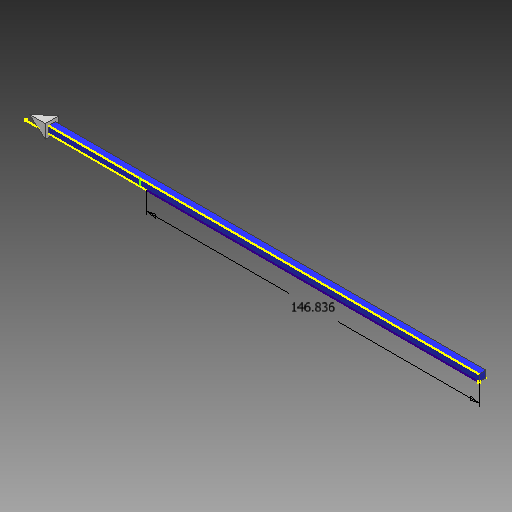
# Autodesk Inventor part: blueStick
Saved by Autodesk Inventor 2018.2 (Build 222227000, 227)
## iProperties
Created: 2018-04-12
Part Number: blueStick
Material: Generisch
Document SubType Name: Modeling
Designer: Nick Koch
Density: 1 g/cm^3
Appearance: Vorgabe
Author: Nick Koch
Autodesk Inventor part; units mm, degrees
ref_plane "YZ Plane" through (0, 0, 0) normal (1, 0, 0) x (0, 1, 0)
ref_plane "XZ Plane" through (0, 0, 0) normal (0, 1, 0) x (-1, 0, 0)
ref_plane "XY Plane" through (0, 0, 0) normal (0, 0, 1) x (1, 0, 0)
sketch "Skizze1" plane through (0, 0, 0) normal (0, 0, 1) x (1, 0, 0)
  line L0 (0, 0) -> (200, 0)
  line L1 (200, 0) -> (200, 3)
  line L2 (200, 3) -> (0, 3)
  line L3 (0, 3) -> (0, 0)
  dimension "d0" = 200
  dimension "d1" = 3
  constraints: 8 end point, 2 parallel, 1 horizontal, 1 perpendicular
  measures "d0" distance of L2.end L1.end
  measures "d1" distance of L1.end L0.end
extrude "Extrusion1" add sketch "Skizze1" along normal blind 3
sketch "Skizze2" plane through (200, 0, 0) normal (1, 0, 0) x (0, 0, -1)
  point P0 (0, 0)
sketch "Skizze3" plane through (0, 0, 0) normal (0, -1, 0) x (1, 0, 0)
  line L0 (0, 0) -> (200, 0) projected
  line L1 (200, 0) -> (53.164, 0)
  dimension "d4" = 146.836
  constraints: 2 end point, 1 point on line
  measures "d4" distance of L0.end L1.end
sketch "Skizze4" plane through (10, 0, 0) normal (-1, 0, 0) x (0, 0, 1)
  line L0 (0, 3) -> (3, 3) projected
  line L1 (0, 0) -> (3, 3)
  line L2 (3, 3) -> (0, 3)
  line L3 (0, 3) -> (3, 0)
  line L4 (-1.5, -1.5) -> (4.5, -1.5)
  line L5 (4.5, -1.5) -> (4.5, 4.5)
  line L6 (4.5, 4.5) -> (-1.5, 4.5)
  line L7 (-1.5, 4.5) -> (-1.5, -1.5)
  line L8 (-1.5, -1.5) -> (4.5, 4.5) construction
  line L9 (4.5, -1.5) -> (-1.5, 4.5) construction
  point P0 (1.5, 1.5)
  dimension "d14" = 6
  dimension "d15" = 6
  constraints: 18 end point, 3 equal length, 3 midpoint, 2 perpendicular, 1 horizontal
  measures "d14" distance of L6.end L5.end
  measures "d15" distance of L5.end L4.end
extrude "Extrusion2" add sketch "Skizze4" along normal blind 10 contours L0 L1 L3 | L7 L6 L5 L4
chamfer "Fase1" distance 2.99 distance2 10 1 edges at (0, 1.5, -1.5) measured on face at (0, 2.5, 0.5)
chamfer "Fase2" distance 2.99 distance2 10 1 edges at (0, 1.5, 4.5) measured on face at (0, 2.5, 2.493)
chamfer "Fase3" distance 2.99 distance2 10 1 edges at (0, -1.5, 1.5) measured on face at (0, 0.5, 1.5035)
chamfer "Fase4" distance 2.99 distance2 10 1 edges at (0, 4.5, 1.5) measured on face at (0, 3.4965, 1.4965)
sketch "Skizze9" plane through (10, 0, 0) normal (0, -1, 0) x (1, 0, 0)
  line L0 (0, 3) -> (190, 3) projected
  line L1 (40.0497, 3) -> (40.0497, 0)
  line L2 (0, 0) -> (190, 0) projected
  point P0 (-10, 0)
  constraints: 2 end point, 2 point on line, 1 vertical
sketch "Skizze10" plane through (0, 0, 0) normal (0, 0, -1) x (-1, 0, 0)
  line L0 (-200, 3) -> (-10, 3) projected
  line L1 (-51.2532, 3) -> (-50.0501, 0)
  line L2 (-10, 0) -> (-200, 0) projected
  point P0 (0, 0)
  constraints: 2 end point, 2 point on line
